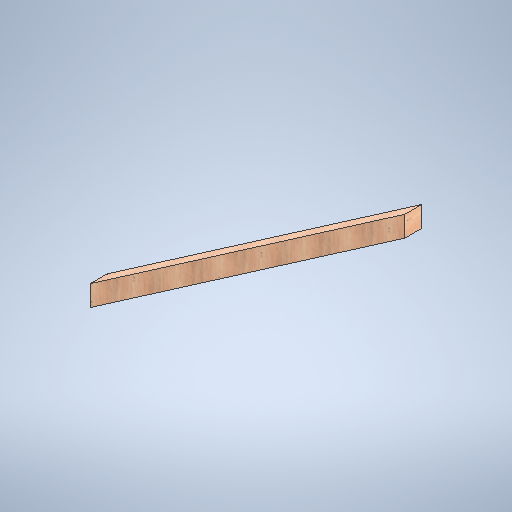
# Autodesk Inventor part: 4x4xigiveup
Saved by Autodesk Inventor 2025 (Build 290162000, 162)
## iProperties
Created: 2024-08-18
Part Number: 4x4xigiveup
Material: Generic
Document SubType Name: Modeling
Designer: Cupri
Density: 1 g/cm^3
Appearance: Default
Author: Cupri
Autodesk Inventor part; units mm, degrees
ref_plane "YZ Plane" through (0, 0, 0) normal (1, 0, 0) x (0, 1, 0)
ref_plane "XZ Plane" through (0, 0, 0) normal (0, 1, 0) x (-1, 0, 0)
ref_plane "XY Plane" through (0, 0, 0) normal (0, 0, 1) x (1, 0, 0)
sketch "Sketch1" plane through (0, 0, 0) normal (0, 0, 1) x (1, 0, 0)
  line L0 (-912.8603, -609.7877) -> (967.9043, 689.8069)
  line L1 (967.9043, 689.8069) -> (1025.6617, 606.2207) construction
  line L2 (967.7522, 566.2057) -> (-913.0123, -733.3889)
  line L3 (-912.8603, -609.7877) -> (-913.0123, -733.3889)
  line L4 (967.9043, 689.8069) -> (967.7522, 566.2057)
  line L5 (-912.8603, -609.7877) -> (-913.0123, -733.3889)
  point P0 (0, 0)
  point P1 (1018.7042, 689.7444)
  dimension "d2" = 101.6
  dimension "d3" = 90
  constraints: 12 end point, 1 perpendicular
  measures "d2" distance of L0.end L1.end
  measures "d3" angle of L1 L2
extrude "Extrusion1" add sketch "Sketch1" along normal blind 101.6
body "Solid1"
